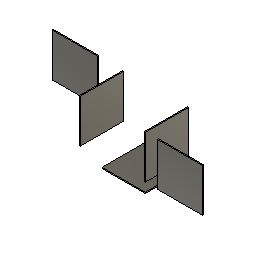
3rdLesson(MoveAndCopyCommand) (v2~recovered) (Autodesk Fusion 360 design; units mm, degrees)
Autodesk Fusion 360 part; units mm, degrees
sketch "Sketch1" plane through (0, 0, 0) normal (1, 0, 0) x (0, 1, 0)
  line L0 (25, 10) -> (125, 10)
  line L1 (125, 10) -> (125, 110)
  line L2 (125, 110) -> (25, 110)
  line L3 (25, 110) -> (25, 10)
  dimension "d1" = 100
  dimension "d2" = 100
  constraint horizontal L0
  constraint vertical L1
  constraint horizontal L2
  constraint vertical L3
  measures "d1" distance of L0.start L0.end
  measures "d2" distance of L0.start L2.end
extrude "Extrude1" add sketch "Sketch1" along normal blind 2.5 makes body 1
copy_body "CopyPasteBodies1" bodies 1 makes body 2
move_body "Move1" bodies 2 to x (1, 0, 0) y (0, 1, 0) z (0, 0, 1) at (0, 0, 0)
move_face "MoveFace1" by (0, 130, 0) 1 faces at (2.5, 58.3333, 76.6667) on bodies 2
move_body "Move2" bodies 1 to x (1, 0, 0) y (0, 1, 0) z (0, 0, 1) at (-70, 0, 70)
copy_body "CopyPasteBodies2" bodies 2 makes body 3
move_body "Move3" bodies 3 to x (1, 0, 0) y (0, 1, 0) z (0, 0, 1) at (0, 0, 0)
move_body "Move4" bodies 3 to x (1, 0, 0) y (0, 1, 0) z (0, 0, 1) at (52.1607, 58.709, 0)
move_body "Move5" bodies 2 to x (0, 0, -1) y (0, 1, 0) z (1, 0, 0) at (-67.0822, 0, 72.0822)
move_body "Move6" bodies 1 to x (1, 0, 0) y (0, 1, 0) z (0, 0, 1) at (10.4178, 0, -7.9178)
move_body "Move7" bodies 2 to x (1, 0, 0) y (0, 1, 0) z (0, 0, 1) at (0, 0, 2.5)
move_body "Move8" bodies 3 to x (1, 0, 0) y (0, 1, 0) z (0, 0, 1) at (-9.2429, -58.709, 64.5822)
move_body "Move9" bodies 3 to x (1, 0, 0) y (0, 1, 0) z (0, 0, 1) at (0, 0, -2.5)
sketch "Sketch2" plane through (0, 0, 0) normal (0, 1, 0) x (1, 0, 0)
  line L0 (110, -70) -> (215, -70)
  line L1 (215, -70) -> (215, -170)
  line L2 (215, -170) -> (110, -170)
  line L3 (110, -170) -> (110, -70)
  dimension "d5" = 105
  dimension "d6" = 100
  constraint horizontal L0
  constraint vertical L1
  constraint horizontal L2
  constraint vertical L3
  measures "d5" distance of L0.start L0.end
  measures "d6" distance of L0.start L2.end
extrude "Extrude2" add sketch "Sketch2" along normal blind 2.5 separate body makes body 4
copy_body "CopyPasteBodies3" bodies 4 makes body 5
move_body "Move10" bodies 5 to x (1, 0, 0) y (0, 1, 0) z (0, 0, 1) at (-280, 0, 0)
move_body "Move11" bodies 5 to x (1, 0, 0) y (0, 1, 0) z (0, 0, 1) at (110.4178, 25, 4.5822)
move_body "Move12" bodies 4 to x (1, 0, 0) y (0, 1, 0) z (0, 0, 1) at (-160, 140, 120)
move_body "Move13" bodies 4 to x (1, 0, 0) y (0, 1, 0) z (0, 0, 1) at (-9.5822, -17.5, -115.4178)
move_body "Move14" bodies 3 to x (1, 0, 0) y (0, 1, 0) z (0, 0, 1) at (0, 0, 110)
move_body "Move15" bodies 3 to x (1, 0, 0) y (0, 1, 0) z (0, 0, 1) at (-2.5, 0, -107.5)
move_body "Move16" bodies 5 to x (1, 0, 0) y (0, 1, 0) z (0, 0, 1) at (130, 0, 0)
move_body "Move17" bodies 4 to x (1, 0, 0) y (0, 1, 0) z (0, 0, 1) at (-140, 0, 0)
move_body "Move18" bodies 2 to x (1, 0, 0) y (0, 1, 0) z (0, 0, 1) at (0, 0, -20)
move_body "Move19" bodies 4 to x (1, 0, 0) y (0, 1, 0) z (0, 0, 1) at (-70, 0, 0)
move_body "Move20" bodies 1 to x (1, 0, 0) y (0, 1, 0) z (0, 0, 1) at (-50, 0, 0)
